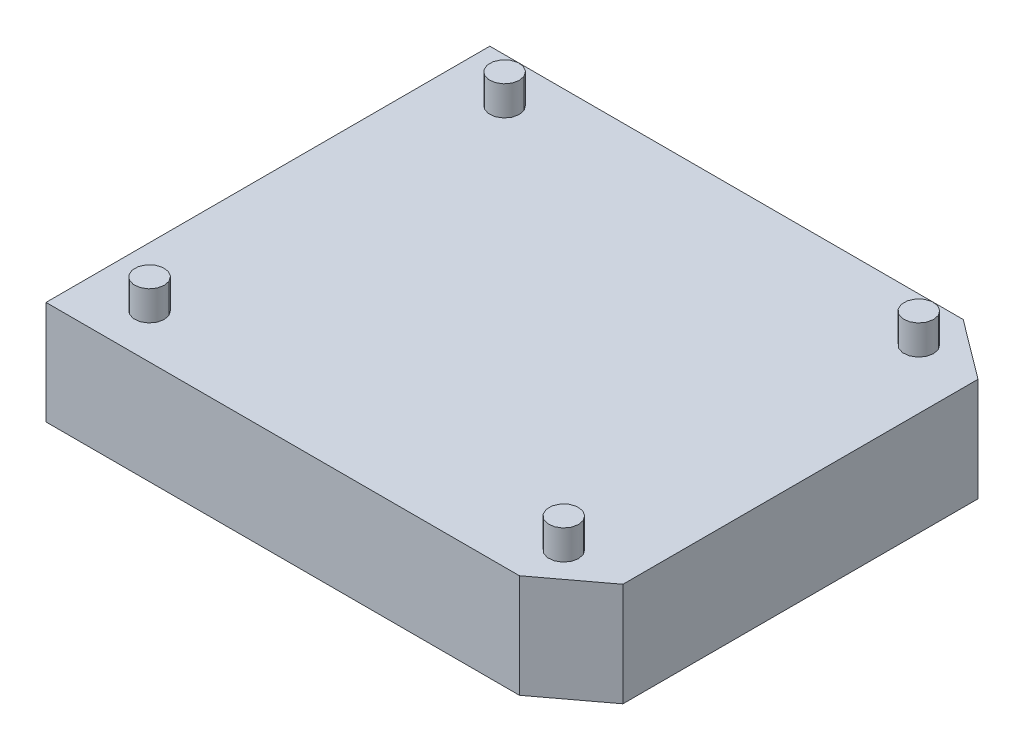
# Autodesk Inventor part: Body Base
Saved by Autodesk Inventor 2016 (Build 200138000, 138)
## iProperties
Created: 2015-09-15
Part Number: Body Base
Material: Aluminum 6061
Document SubType Name: Modeling
Designer: rossmosier
Density: 2.7 g/cm^3
Appearance: Aluminum - Flat
Author: rossmosier
Autodesk Inventor part; units mm, degrees
ref_plane "YZ Plane" through (0, 0, 0) normal (1, 0, 0) x (0, 1, 0)
ref_plane "XZ Plane" through (0, 0, 0) normal (0, 1, 0) x (-1, 0, 0)
ref_plane "XY Plane" through (0, 0, 0) normal (0, 0, 1) x (1, 0, 0)
sketch "Sketch1" plane through (0, 0, 0) normal (0, 1, 0) x (-1, 0, 0)
  line L0 (0, 0) -> (-457.2, 0) construction
  line L1 (-457.2, -457.2) -> (0, -457.2) construction
  line L2 (0, -457.2) -> (0, 0) construction
  line L3 (0, 0) -> (0, -38.1) construction
  line L4 (0, -457.2) -> (0, -419.1) construction
  line L5 (0, -38.1) -> (0, -371.3712)
  line L6 (-457.2, -76.2) -> (-457.2, -381)
  line L7 (0, -371.3712) -> (0, -419.1)
  line L8 (-406.4, -38.1) -> (-457.2, -76.2)
  line L9 (-406.4, -419.1) -> (-457.2, -381)
  line L10 (-457.2, 0) -> (-457.2, -38.1) construction
  line L11 (-457.2, -76.2) -> (-457.2, -457.2) construction
  line L12 (-444.5, -82.55) -> (-444.5, -374.65)
  line L13 (-444.5, -374.65) -> (-402.1667, -406.4)
  line L14 (-12.7, -406.4) -> (-12.7, -371.3712)
  line L15 (-12.7, -371.3712) -> (-12.7, -50.8)
  line L16 (-402.1667, -50.8) -> (-444.5, -82.55)
  line L17 (-444.5, -82.55) -> (-444.5, -374.65)
  line L18 (-444.5, -374.65) -> (-402.1667, -406.4)
  line L19 (-12.7, -406.4) -> (-12.7, -371.3712)
  line L20 (-12.7, -371.3712) -> (-12.7, -50.8)
  line L21 (-402.1667, -50.8) -> (-444.5, -82.55)
  line L22 (-444.5, -82.55) -> (-444.5, -374.65)
  line L23 (-12.7, -406.4) -> (-12.7, -50.8)
  line L24 (-444.5, -82.55) -> (-444.5, -374.65)
  line L25 (-402.1667, -50.8) -> (-12.7, -50.8)
  line L26 (-406.4, -38.1) -> (0, -38.1)
  line L27 (-406.4, -419.1) -> (0, -419.1)
  line L28 (-402.1667, -406.4) -> (-12.7, -406.4)
  dimension "d0" = 457.2
  dimension "d1" = 457.2
  dimension "d12" = 12.7
  dimension "d13" = 12.7
  constraints: 58 end point, 6 parallel, 3 collinear, 3 point on line, 2 horizontal, 2 perpendicular, 2 vertical, 4 other
  measures "d0" distance of L1.end L1.start
  measures "d1" distance of L1.start L0.end
  measures "d12" distance between parallel lines of L8 L16
  measures "d13" distance between parallel lines of L8 L21
extrude "Extrusion1" add sketch "Sketch1" along normal blind 88.9 contours L5 L7 L27 L9 L6 L8 L26 | L16 L25 L15 L14 L28 L13 L12
sketch "Sketch2" plane through (0, 0, 0) normal (0, -1, 0) x (1, 0, 0)
  line L0 (0, -38.1) -> (0, -419.1) projected
  line L1 (406.4, -419.1) -> (457.2, -381) projected
  line L2 (457.2, -381) -> (457.2, -76.2) projected
  line L3 (457.2, -76.2) -> (406.4, -38.1) projected
  line L4 (402.1667, -50.8) -> (444.5, -82.55)
  line L5 (444.5, -82.55) -> (444.5, -374.65)
  line L6 (444.5, -374.65) -> (402.1667, -406.4)
  line L7 (402.1667, -406.4) -> (368.3, -406.4)
  line L8 (368.3, -406.4) -> (368.3, -330.2)
  line L9 (368.3, -330.2) -> (88.9, -330.2)
  line L10 (88.9, -330.2) -> (88.9, -374.65)
  line L11 (88.9, -374.65) -> (46.5667, -406.4)
  line L12 (46.5667, -406.4) -> (12.7, -406.4)
  line L13 (12.7, -406.4) -> (12.7, -50.8)
  line L14 (12.7, -50.8) -> (46.5667, -50.8)
  line L15 (46.5667, -50.8) -> (88.9, -82.55)
  line L16 (88.9, -82.55) -> (88.9, -127)
  line L17 (88.9, -127) -> (368.3, -127)
  line L18 (368.3, -127) -> (368.3, -50.8)
  line L19 (368.3, -50.8) -> (402.1667, -50.8)
  line L20 (0, -419.1) -> (406.4, -419.1) projected
  line L21 (406.4, -38.1) -> (0, -38.1) projected
  point P0 (0, 0)
  dimension "d14" = 12.7
  constraints: 32 end point, 2 other
  measures "d14" distance between parallel lines of L3 L4
extrude "Extrusion2" cut sketch "Sketch2" against normal blind 76.2 contours L4 L5 L6 L7 L8 L9 L10 L11 L12 L13 L14 L15 L16 L17 L18 L19
sketch "Sketch3" plane through (0, 88.9, 0) normal (0, 1, 0) x (1, 0, 0)
  line L0 (0, 419.1) -> (0, 38.1) projected
  line L1 (406.4, 38.1) -> (457.2, 76.2) projected
  line L2 (457.2, 76.2) -> (457.2, 381) projected
  line L3 (457.2, 381) -> (406.4, 419.1) projected
  circle A0 centre (50.8, 76.2) radius 12.7
  circle A1 centre (50.8, 381) radius 12.7
  circle A2 centre (406.4, 381) radius 12.7
  circle A3 centre (406.4, 76.2) radius 12.7
  line L4 (0, 38.1) -> (406.4, 38.1) projected
  line L5 (406.4, 419.1) -> (0, 419.1) projected
  point P0 (0, 0)
  dimension "d17" = 25.4
  dimension "d18" = 25.4
  dimension "d19" = 25.4
  dimension "d20" = 25.4
  constraints: 4 centre point
  measures "d17" diameter of A0
  measures "d18" diameter of A1
  measures "d19" diameter of A2
  measures "d20" diameter of A3
extrude "Extrusion3" add sketch "Sketch3" along normal blind 25.4 contours A0 | A1 | A2 | A3
body "Solid1"
